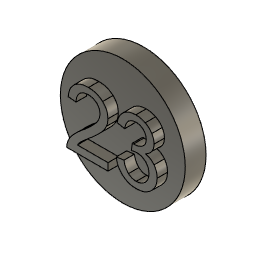
정보관 본체 v27 (Autodesk Fusion 360 archive; units mm, degrees)
design "정보관 번호 23"
Autodesk Fusion 360 part; units mm, degrees
sketch "스케치2" plane through (0, 0, 0) normal (0, 1, 0) x (1, 0, 0)
  circle A0 centre (0, 0) radius 3
  line L0 (-2.2753, 2.0091) -> (2.2279, 2.0091) construction
  line L1 (2.2279, 2.0091) -> (2.2279, -1.9552) construction
  line L2 (2.2279, -1.9552) -> (-2.2753, -1.9552) construction
  line L3 (-2.2753, -1.9552) -> (-2.2753, 2.0091) construction
  dimension "d4" = 6
  dimension "d5" = 3
  text T0 "23" font "Arial" height 3 align centre middle in box 4.5032 x 3.9643 at (-2.2753, 2.0091) x (1, 0) y (0, -1) spacing 1 kerned
  constraint coincident A0.centre origin
  constraint coincident A0
  measures "d4" diameter of A0
extrude "돌출1" add sketch "스케치2" along normal blind 1
extrude "돌출2" add sketch "스케치2" against normal blind 0.5 text T0
